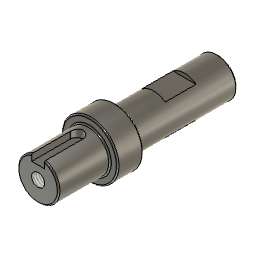
04 (Autodesk Fusion 360 design; units mm, degrees)
Autodesk Fusion 360 part; units mm, degrees
sketch "Sketch1" plane through (0, 0, 0) normal (1, 0, 0) x (0, 1, 0)
  line L0 (-35, 0) -> (35, 0)
  line L1 (-35, 0) -> (-35, 8)
  line L2 (-35, 8) -> (-15, 8)
  line L3 (-15, 8) -> (-15, 11)
  line L4 (-15, 11) -> (-5, 11)
  line L5 (-5, 11) -> (-5, 7.5)
  line L6 (-5, 7.5) -> (35, 7.5)
  line L7 (35, 7.5) -> (35, 0)
  dimension "d8" = 70
  dimension "d9" = 40
  dimension "d10" = 10
  dimension "d11" = 8
  dimension "d12" = 7.5
  dimension "d14" = 11
  constraint horizontal L0
  constraint midpoint origin L0
  constraint perpendicular L0 L1
  constraint perpendicular L1 L2
  constraint perpendicular L2 L3
  constraint perpendicular L3 L4
  constraint perpendicular L2 L5
  constraint perpendicular L5 L6
  constraint perpendicular L0 L7
  measures "d8" distance of L0.start L0.end
  measures "d9" distance of L5.end L6.end
  measures "d10" distance of L3.end L4.end
  measures "d11" distance of L0.start L1.end
  measures "d12" distance of L0.end L6.end
  measures "d14" distance of L0 L4
revolve "Revolve1" add sketch "Sketch1" angle 360 about axis through (0, -35, 0) along (0, 1, 0)
sketch "Sketch5" plane through (0, 0, 0) normal (1, 0, 0) x (0, 1, 0)
  line L0 (35, 7.5) -> (-5, 7.5)
  line L1 (-5, -7.5) -> (35, -7.5)
  line L2 (10, 7.5) -> (22, 7.5)
  line L3 (22, 7.5) -> (22, 6)
  line L4 (22, 6) -> (10, 6)
  line L5 (10, 6) -> (10, 7.5)
  line L6 (22, -7.5) -> (10, -7.5)
  line L7 (10, -7.5) -> (10, -6)
  line L8 (10, -6) -> (22, -6)
  line L9 (22, -6) -> (22, -7.5)
  dimension "d16" = 15
  dimension "d17" = 12
  dimension "d18" = 1.5
  dimension "d19" = 1.5
  constraint horizontal L2
  constraint vertical L3
  constraint horizontal L4
  constraint vertical L5
  constraint coincident L0 L2.start
  constraint horizontal L6
  constraint vertical L7
  constraint horizontal L8
  constraint vertical L9
  constraint coincident L1 L6.start
  constraint equal L4 L8
  constraint vertical L4.end L7.end
  measures "d16" distance of L0.end L2.start
  measures "d17" distance of L3.end L4.end
  measures "d18" distance of L2.start L4.end
  measures "d19" distance of L6.end L7.end
extrude "Extrude1" cut sketch "Sketch5" along normal through all and the other way through all
ref_plane "WorkPlane1" through (0, -21.8673, 8) normal (0, 0, 1) x (-1, 0, 0)
sketch "Sketch9" plane through (0, -21.8673, 8) normal (0, 0, 1) x (1, 0, 0)
  line L0 (8, -13.1327) -> (-8, -13.1327)
  line L1 (-7.9118, -13.1327) -> (8, -13.1327)
  line L2 (2.5, -13.1327) -> (2.5, 1.8673)
  arc A0 (2.5, 1.8673) -> (-2.5, 1.8673) centre (0, 1.8673) ccw
  line L3 (-2.5, 1.8673) -> (-2.5, -13.1327)
  arc A1 (-2.5, -13.1327) -> (2.5, -13.1327) centre (0, -13.1327) ccw
  line L4 (0, -13.1327) -> (0, 1.8673) construction
  point P0 (0, -13.1327)
  dimension "d23" = 15
  dimension "d24" = 5
  constraint coincident L0 L1.start
  constraint parallel L0 L1
  constraint tangent L2 A0
  constraint tangent A0 L3
  constraint parallel L2 L3
  constraint tangent L3 A1
  constraint tangent L2 A1
  constraint perpendicular L1 L4
  constraint coincident P0 A1.centre
  measures "d23" distance of P0 A0.centre
  measures "d24" diameter of A0
extrude "Extrude2" cut sketch "Sketch9" against normal blind 3
hole "Hole1" at (0, -35, 0) direction (0, 1, 0) diameter 5.035 depth 15 tip angle 118
thread "Thread1" "ISO Metric profile 6.0 M6x1 6H" thread offset 0 thread depth 12
fillet "Fillet1" radius 0.5 6 edges at (0, -35, -8) (-10.2556, -15, 3.9778) (-7.4586, -15, 2.8929) (-10.2556, -5, 3.9778) (-6.9925, -5, 2.7121) (-6.9925, 35, 2.7121)
sketch "Sketch8" plane through (0, 0, 0) normal (0, 0, 1) x (1, 0, 0)
sketch "Sketch7" plane through (0, -21.8673, 8) normal (0, 0, 1) x (1, 0, 0)
  line L0 (8, -13.1327) -> (-8, -13.1327)
  line L1 (-8.1705, -13.1327) -> (8, -13.1327)
  constraint parallel L0 L1
